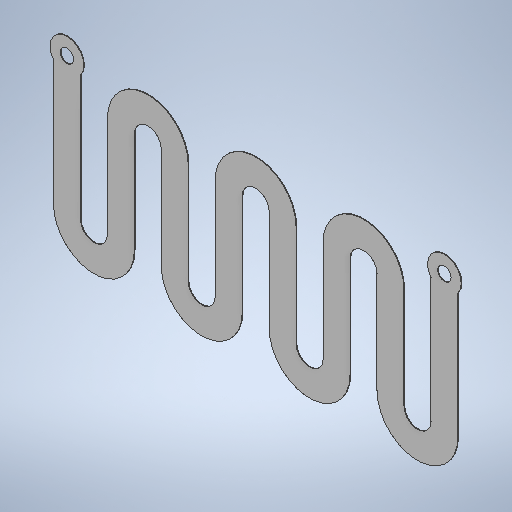
# Autodesk Inventor part: sensor-0002-001
Saved by Autodesk Inventor 2025.2 (Build 292293000, 293)
## iProperties
Created: 2025-01-26
Part Number: sensor-0002-001
Material: Generic
Document SubType Name: Modeling
Designer: kenne
Density: 1 g/cm^3
Appearance: Default
Author: kenne
Autodesk Inventor part; units mm, degrees
ref_plane "YZ Plane" through (0, 0, 0) normal (1, 0, 0) x (0, 1, 0)
ref_plane "XZ Plane" through (0, 0, 0) normal (0, 1, 0) x (-1, 0, 0)
ref_plane "XY Plane" through (0, 0, 0) normal (0, 0, 1) x (1, 0, 0)
sketch "Sketch3" plane through (0, 0, 0) normal (0, 0, 1) x (1, 0, 0)
  circle A0 centre (-2800, 0) radius 250 construction
  line L0 (-2800, 0) -> (-2800, -2000) construction
  line L1 (-3000, -150) -> (-3000, -2000)
  line L2 (-2600, -150) -> (-2600, -2000)
  circle A1 centre (-2400, -2000) radius 200 construction
  arc A2 (-2600, -2000) -> (-2200, -2000) centre (-2400, -2000) ccw
  circle A3 centre (-2400, -2000) radius 600 construction
  arc A4 (-3000, -2000) -> (-1800, -2000) centre (-2400, -2000) ccw
  line L3 (-2200, -2000) -> (-2200, -500)
  line L4 (-1800, -2000) -> (-1800, -500)
  circle A5 centre (-1600, -500) radius 200 construction
  arc A6 (-1400, -500) -> (-1800, -500) centre (-1600, -500) ccw
  circle A7 centre (-1600, -500) radius 600 construction
  arc A8 (-1000, -500) -> (-2200, -500) centre (-1600, -500) ccw
  line L5 (-1400, -500) -> (-1400, -2000)
  line L6 (-1000, -500) -> (-1000, -2000)
  circle A9 centre (-800, -2000) radius 200 construction
  arc A10 (-1000, -2000) -> (-600, -2000) centre (-800, -2000) ccw
  circle A11 centre (-800, -2000) radius 600 construction
  arc A12 (-1400, -2000) -> (-200, -2000) centre (-800, -2000) ccw
  line L7 (-600, -2000) -> (-600, -500)
  line L8 (-200, -2000) -> (-200, -500)
  circle A13 centre (0, -500) radius 200 construction
  arc A14 (200, -500) -> (-200, -500) centre (0, -500) ccw
  circle A15 centre (0, -500) radius 600 construction
  arc A16 (600, -500) -> (-600, -500) centre (0, -500) ccw
  line L9 (200, -500) -> (200, -2000)
  line L10 (600, -500) -> (600, -2000)
  circle A17 centre (800, -2000) radius 200 construction
  arc A18 (600, -2000) -> (1000, -2000) centre (800, -2000) ccw
  circle A19 centre (800, -2000) radius 600 construction
  arc A20 (200, -2000) -> (1400, -2000) centre (800, -2000) ccw
  line L11 (1000, -2000) -> (1000, -500)
  line L12 (1400, -2000) -> (1400, -500)
  circle A21 centre (1600, -500) radius 200 construction
  arc A22 (1800, -500) -> (1400, -500) centre (1600, -500) ccw
  circle A23 centre (1600, -500) radius 600 construction
  arc A24 (2200, -500) -> (1000, -500) centre (1600, -500) ccw
  line L13 (1800, -500) -> (1800, -2000)
  line L14 (2200, -500) -> (2200, -2000)
  circle A25 centre (2400, -2000) radius 200 construction
  arc A26 (2200, -2000) -> (2600, -2000) centre (2400, -2000) ccw
  circle A27 centre (2400, -2000) radius 600 construction
  arc A28 (1800, -2000) -> (3000, -2000) centre (2400, -2000) ccw
  line L15 (2600, -2000) -> (2600, -150)
  line L16 (3000, -2000) -> (3000, -150)
  circle A29 centre (2800, 0) radius 250 construction
  line L17 (-2800, 0) -> (2800, 0) construction
  circle A30 centre (-2800, 0) radius 100
  circle A31 centre (2800, 0) radius 100
  arc A32 (-2600, -150) -> (-3000, -150) centre (-2800, 0) ccw
  arc A33 (3000, -150) -> (2600, -150) centre (2800, 0) ccw
  point P0 (0, 0)
  point P1 (0, 0)
  point P2 (0, 0)
  dimension "d52" = 500
  dimension "d40" = 500
  dimension "d41" = 2000
  dimension "d42" = 200
  dimension "d44" = 400
  dimension "d45" = 1500
  dimension "d46" = 400
  dimension "d47" = 400
  dimension "d48" = 400
  dimension "d49" = 400
  dimension "d50" = 400
  dimension "d51" = 400
  dimension "d53" = 200
  dimension "d54" = 200
  constraints: 63 point on circle, 36 end point, 34 tangent, 33 centre point, 23 horizontal alignment, 17 vertical, 14 parallel, 12 coincident, 2 concentric, 1 horizontal, 1 midpoint, 4 other
  measures "d40" diameter of A0
  measures "d41" distance of L0.start L0.end
  measures "d42" distance between parallel lines of L1 L0
  measures "d44" diameter of A1
  measures "d45" distance of L3.start L3.end
  measures "d46" diameter of A5
  measures "d47" diameter of A9
  measures "d48" diameter of A13
  measures "d49" diameter of A17
  measures "d50" diameter of A21
  measures "d51" diameter of A25
  measures "d53" diameter of A30
  measures "d54" diameter of A31
extrude "Extrusion2" add sketch "Sketch3" along normal blind 10
body "Solid2"
